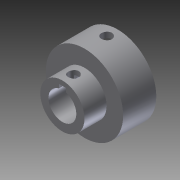
# Autodesk Inventor part: sprocket hub adaptor
Saved by Autodesk Inventor 2012 (Build 160160000, 160)
## iProperties
Created: 2013-07-25
Part Number: sprocket hub adaptor
Material: Default
Document SubType Name: Modeling
Designer: Bryce
Density: 1 g/cm^3
Author: Bryce
Autodesk Inventor part; units mm, degrees
ref_plane "YZ Plane" through (0, 0, 0) normal (1, 0, 0) x (0, 1, 0)
ref_plane "XZ Plane" through (0, 0, 0) normal (0, 1, 0) x (-1, 0, 0)
ref_plane "XY Plane" through (0, 0, 0) normal (0, 0, 1) x (1, 0, 0)
sketch "Sketch1" plane through (0, 0, 0) normal (0, 0, 1) x (1, 0, 0)
  circle A0 centre (0, 0) radius 9.525
  circle A1 centre (0, 0) radius 11.1125
  circle A2 centre (0, 0) radius 4
  circle A3 centre (0, 0) radius 6.35
  line L0 (-1, 3) -> (1, 3)
  line L1 (1, 3) -> (1, 5)
  line L2 (1, 5) -> (-1, 5)
  line L3 (-1, 5) -> (-1, 3)
  dimension "d0" = 19.05
  dimension "d1" = 22.225
  dimension "d2" = 8
  dimension "d3" = 12.7
  dimension "d15" = 2
  dimension "d16" = 2
  dimension "d17" = 1
  dimension "d18" = 5
  constraints: 8 end point, 4 centre point, 4 coincident, 2 parallel, 1 horizontal, 1 perpendicular
  measures "d0" diameter of A0
  measures "d1" diameter of A1
  measures "d2" diameter of A2
  measures "d3" diameter of A3
  measures "d15" distance of L1.end L2.end
  measures "d16" distance of L2.end L0.start
  measures "d17" distance from line of L1 point (0, 0)
  measures "d18" distance from line of L2 point (0, 0)
extrude "Extrusion1" add sketch "Sketch1" along normal blind 3.175 contours A0 | A1 | A2 L3 L2 L1 | A3
extrude "Extrusion2" add sketch "Sketch1" along normal blind 9.525 contours A3
extrude "Extrusion3" add sketch "Sketch1" against normal blind 6.35 contours A1
sketch "Sketch2" plane through (0, 0, 0) normal (0, 1, 0) x (-1, 0, 0)
  circle A0 centre (0, 6.35) radius 1.5
  circle A1 centre (0, -3.175) radius 1.5
  line L0 (-9.525, 0) -> (9.525, 0) projected
  line L1 (-4, 9.525) -> (4, 9.525) projected
  point P0 (0, 0)
  point P1 (0, 0)
  dimension "d10" = 3
  dimension "d11" = 3.175
  dimension "d12" = 3.175
  constraints: 2 centre point, 2 vertical alignment, 1 equal radius, 1 midpoint
  measures "d10" diameter of A0
  measures "d11" distance from line of A1.centre L0
  measures "d12" distance from line of L1 A0.centre
extrude "Extrusion4" cut sketch "Sketch2" along normal through all
equation "\"d16\" = d15"
equation "\"d17\" = 0.5 * d15"
equation "\"d18\" = 0.5 * d2 + d17"
body "Solid1"
